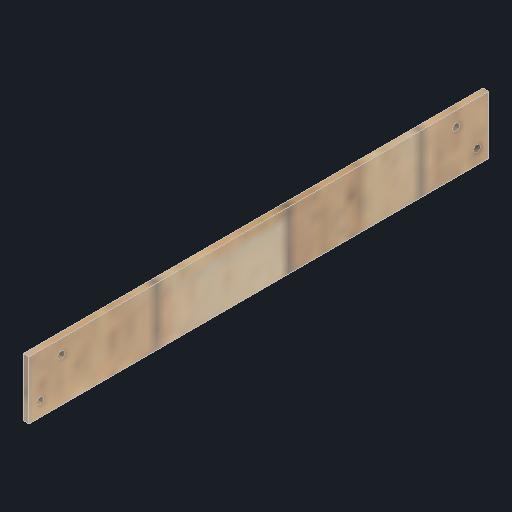
# Autodesk Inventor part: Side_Wall_Riner
Saved by Autodesk Inventor 2026.3 (Build 303398000, 398)
## iProperties
Created: 2026-09-07
Part Number: Side_Wall_Riner
Material: 木材 (カエデ材)
Document SubType Name: Modeling
Designer: takuya
Density: 0.67 g/cm^3
Appearance: ナチュラル カエデ材 - 光沢 濃い着色
Author: takuya
Autodesk Inventor part; units mm, degrees
ref_plane "YZ Plane" through (0, 0, 0) normal (1, 0, 0) x (0, 1, 0)
ref_plane "XZ Plane" through (0, 0, 0) normal (0, 1, 0) x (-1, 0, 0)
sketch "スケッチ1" plane through (0, 0, 0) normal (0, 0, 1) x (1, 0, 0)
  line L0 (-53.8577, -21) -> (53.8577, -21) projected
  line L1 (53.8577, -21) -> (53.8577, -19.5) projected
  line L2 (53.8577, -19.5) -> (45.423, -16.1743) projected
  line L3 (45.423, -16.1743) -> (44.506, -18.5) projected
  line L4 (44.506, -18.5) -> (-49.7747, 18.6743) projected
  line L5 (-49.7747, 18.6743) -> (-48.8577, 21) projected
  line L6 (-48.8577, 21) -> (-53.8577, 21) projected
  line L7 (-53.8577, 21) -> (-53.8577, -21) projected
  line L8 (-42.0411, 10.2503) -> (14.7433, -12.1394) projected
  arc A0 (14.0097, -16) -> (14.7433, -12.1394) centre (14.0097, -14) ccw projected
  line L9 (14.0097, -16) -> (-42.7747, -16) projected
  arc A1 (-44.7747, -14) -> (-42.7747, -16) centre (-42.7747, -14) ccw projected
  line L10 (-44.7747, -14) -> (-44.7747, 8.3897) projected
  arc A2 (-42.0411, 10.2503) -> (-44.7747, 8.3897) centre (-42.7747, 8.3897) ccw projected
  arc A3 (-76.8577, -9) -> (-66.8577, -11) centre (-66.8577, 15) ccw projected
  arc A4 (-86.8577, -11) -> (-76.8577, -9) centre (-86.8577, 15) ccw projected
  line L11 (-86.8577, -13) -> (-86.8577, -11) projected
  line L12 (-86.8577, -13) -> (-66.8577, -13) projected
  line L13 (-66.8577, -21) -> (-66.8577, -13) projected
  line L14 (-53.8577, -21) -> (-66.8577, -21) projected
  line L15 (-53.8577, -4) -> (-53.8577, -21) projected
  line L16 (-56.8577, -4) -> (-53.8577, -4) projected
  line L17 (-56.8577, -11) -> (-56.8577, -4) projected
  line L18 (-66.8577, -11) -> (-56.8577, -11) projected
  line L19 (-53.8577, 21) -> (-56.3577, 21)
  line L20 (-56.3577, 21) -> (-56.3577, -4)
  line L21 (-56.3577, -4) -> (-53.8577, -4)
  line L22 (-53.8577, -4) -> (-53.8577, 21)
  point P0 (0, 0)
  dimension "d0" = 2.5
  constraints: 8 end point, 2 parallel, 1 horizontal, 1 perpendicular, 1 point on line
  measures "d0" distance of L6.end L19.end
ref_plane "作業平面1" through (-53.8577, -21, -198) normal (0, 0, -1) x (0, 1, 0)
extrude "押し出し1" add sketch "スケッチ1" against normal up to surface (198 mm away) contours L16 L20 L19 L7
sketch "スケッチ2" plane through (-56.3577, -4, 0) normal (-1, 0, 0) x (0, 0, 1)
  line L0 (-198, 25) -> (-198, 0) projected
  line L1 (0, 0) -> (-198, 0) projected
  line L2 (0, 25) -> (0, 0) projected
  line L3 (0, 25) -> (-198, 25) projected
  line L4 (-198, -10) -> (-188, -10) projected
  line L5 (-198, 12.3897) -> (-198, -10) projected
  line L6 (-188, 12.3897) -> (-198, 12.3897) projected
  line L7 (-188, -10) -> (-188, 12.3897) projected
  line L8 (-10, -10) -> (0, -10) projected
  line L9 (-10, 12.3897) -> (-10, -10) projected
  line L10 (0, 12.3897) -> (-10, 12.3897) projected
  line L11 (0, -10) -> (0, 12.3897) projected
  line L12 (0, 0) -> (-198, 0) projected
  line L13 (-198, 12.3897) -> (-188, 12.3897)
  line L14 (-188, 12.3897) -> (-188, 0)
  line L15 (-188, 0) -> (-198, 0)
  line L16 (-198, 0) -> (-198, 12.3897)
  line L17 (0, 12.3897) -> (-10, 12.3897)
  line L18 (-10, 12.3897) -> (-10, 0)
  line L19 (-10, 0) -> (0, 0)
  line L20 (0, 0) -> (0, 12.3897)
  circle A0 centre (-193, 6.1949) radius 1.5
  circle A1 centre (-5, 6.1949) radius 1.5
  point P0 (0, 4)
  dimension "d3" = 3
  dimension "d4" = 3
  constraints: 16 end point, 4 parallel, 4 point on line, 2 centre point, 2 horizontal, 2 perpendicular
  measures "d3" diameter of A0
  measures "d4" diameter of A1
extrude "押し出し2" cut sketch "スケッチ2" against normal blind 2.5 contours A0 | A1
sketch "スケッチ3" plane through (-56.3577, -4, 0) normal (-1, 0, 0) x (0, 0, 1)
  circle A0 centre (-184, 18.6743) radius 1.5 projected
  circle A1 centre (-14, 18.6743) radius 1.5 projected
  point P0 (0, 4)
extrude "押し出し3" cut sketch "スケッチ3" against normal blind 2.5
